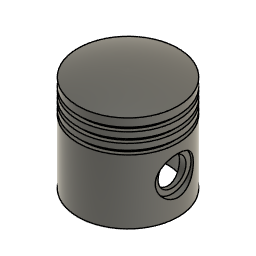
Piston_ (Autodesk Fusion 360 design; units mm, degrees)
Autodesk Fusion 360 part; units mm, degrees
sketch "Sketch1" plane through (0, 0, 0) normal (0, 1, 0) x (1, 0, 0)
  line L0 (0, 0) -> (0, -408.4277) construction
  line L1 (0, -660.4) -> (0, -355.6)
  line L2 (0, -355.6) -> (254, -355.6)
  line L3 (254, -355.6) -> (254, 0)
  line L4 (254, 0) -> (317.5, 0)
  line L5 (317.5, 0) -> (317.5, -406.4)
  line L6 (317.5, -406.4) -> (292.1, -406.4)
  line L7 (292.1, -406.4) -> (292.1, -431.8)
  line L8 (292.1, -431.8) -> (317.5, -431.8)
  line L9 (317.5, -431.8) -> (317.5, -469.9)
  line L10 (317.5, -469.9) -> (292.1, -469.9)
  line L11 (292.1, -469.9) -> (292.1, -495.3)
  line L12 (292.1, -495.3) -> (317.5, -495.3)
  line L13 (317.5, -495.3) -> (317.5, -533.4)
  line L14 (317.5, -533.4) -> (292.1, -533.4)
  line L15 (292.1, -533.4) -> (292.1, -558.8)
  line L16 (292.1, -558.8) -> (317.5, -558.8)
  line L17 (317.5, -558.8) -> (317.5, -609.6)
  arc A0 (0, -660.4) -> (317.5, -609.6) centre (0, 357.1875) ccw
  line L18 (0, -660.4) -> (-298.2009, -660.4) construction
  dimension "d1" = 508
  dimension "d2" = 635
  dimension "d3" = 355.6
  dimension "d4" = 406.4
  dimension "d5" = 25.4
  dimension "d6" = 25.4
  dimension "d7" = 38.1
  dimension "d8" = 50.8
  dimension "d9" = 660.4
  constraint coincident L0.start origin
  constraint vertical L0
  constraint coincident L0 L1.start
  constraint coincident L0 L1.end
  constraint perpendicular L1 L2
  constraint perpendicular L2 L3
  constraint perpendicular L0 L4
  constraint perpendicular L4 L5
  constraint perpendicular L5 L6
  constraint perpendicular L6 L7
  constraint perpendicular L7 L8
  constraint perpendicular L8 L9
  constraint perpendicular L9 L10
  constraint perpendicular L10 L11
  constraint perpendicular L11 L12
  constraint perpendicular L12 L13
  constraint perpendicular L13 L14
  constraint perpendicular L14 L15
  constraint perpendicular L15 L16
  constraint perpendicular L16 L17
  constraint horizontal L0.start L3.end
  constraint vertical L5.end L8.end
  constraint vertical L9.end L12.end
  constraint vertical L13.end L17.end
  constraint equal L7 L11
  constraint equal L11 L15
  constraint equal L9 L13
  constraint vertical L7.end L10.end
  constraint vertical L11.end L14.end
  constraint perpendicular L1 L18
  constraint tangent A0 L18
  measures "d3" distance of L2.end L3.end
  measures "d4" distance of L4.end L5.end
  measures "d5" distance of L5.end L6.end
  measures "d6" distance of L6.end L7.end
  measures "d7" distance of L8.end L9.end
  measures "d8" distance of L16.end L17.end
  measures "d9" distance of L0.start L1.start
revolve "Revolve1" add sketch "Sketch1" angle 360 about axis through (0, 0, 0) along (0, 0, 1)
ref_plane "WorkPlane1" through (317.5, 0, 0) normal (1, 0, 0) x (0, 1, 0)
sketch "Sketch2" plane through (317.5, 0, 0) normal (1, 0, 0) x (0, 1, 0)
  circle A0 centre (0, 228.6) radius 120.65
  dimension "d12" = 241.3
  dimension "d13" = 228.6
  constraint vertical origin A0.centre
  measures "d12" diameter of A0
  measures "d13" distance of origin A0.centre
extrude "Extrude1" cut sketch "Sketch2" against normal blind 38.1
sketch "Sketch3" plane through (279.4, 0, 0) normal (1, 0, 0) x (0, 1, 0)
  circle A0 centre (0, 228.6) radius 120.65
  circle A1 centre (0, 228.6) radius 88.9
  dimension "d16" = 177.8
  constraint concentric A0 A1
  measures "d16" diameter of A1
extrude "Extrude2" cut sketch "Sketch3" against normal blind 127 contours A1
mirror "Mirror1" about plane through (0, 0, 0) normal (1, 0, 0) of "Extrude1", "Extrude2"
